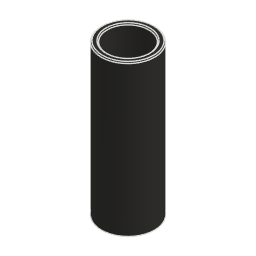
8mm_bearing_adapter_x2 (Autodesk Fusion 360 design; units mm, degrees)
Autodesk Fusion 360 part; units mm, degrees
sketch "Sketch1" plane through (0, 0, 0) normal (0, 1, 0) x (1, 0, 0)
  line L0 (0, 0) -> (0, -55)
  line L1 (0, -55) -> (-9.675, -55)
  line L2 (-9.675, -55) -> (-9.675, 0)
  line L3 (-9.675, 0) -> (0, 0)
  line L4 (-7.5, -55) -> (-7.5, -30.5)
  line L5 (-7.5, 0) -> (-7.5, -24.5)
  line L6 (-7.5, -24.5) -> (0, -24.5)
  line L7 (-7.5, -30.5) -> (0, -30.5)
  line L8 (-7.5, -24.5) -> (-7.5, -30.5)
  line L9 (-5.5, -24.5) -> (-5.5, -30.5)
  dimension "d1" = 19.35
  dimension "d2" = 55
  dimension "d5" = 24.5
  dimension "d6" = 24.5
  dimension "d7" = 15
  dimension "d27" = 2
  constraint coincident L0.start L3.end
  constraint vertical L0
  constraint vertical L2
  constraint horizontal L3
  constraint horizontal L1
  constraint coincident L1 L4.start
  constraint vertical L4
  constraint coincident L3 L5.start
  constraint vertical L5
  constraint coincident L0 L6.end
  constraint coincident L0 L7.end
  constraint horizontal L7
  constraint horizontal L6
  constraint coincident L7 L4.end
  constraint vertical L8
  constraint coincident L4.end L7.start
  constraint coincident L5.end L6.start
  constraint coincident L6 L9.start
  constraint coincident L7 L9.end
  constraint perpendicular L7 L9
  measures "d2" distance of L0.start L0.end
  measures "d5" distance of L5.start L5.end
  measures "d6" distance of L4.start L4.end
  measures "d27" distance of L4.end L9.end
revolve "Revolve1" add sketch "Sketch1" angle 360 about axis through (0, 0, 0) along (0, 0, 1) contours L1 L2 L3 L4 L5 L8 | L6 L7 L8 L9
move_face "OffsetFaces2" offset -0.075 3 faces at (-7.4627, 0.7468, 46.8333) (-7.4907, 0.3738, 16.3333) (-5.4932, 0.2742, 26.5)
chamfer "Chamfer5" distance 0.4 angle 45 2 edges at (7.0624, -2.7392, 55) (-9.0203, 3.4986, 55)
chamfer "Chamfer6" distance 0.2 angle 45 2 edges at (7.0624, -2.7392, 0) (-9.0203, 3.4986, 0)
chamfer "Chamfer7" distance 2 angle 45 2 edges at (5.1977, -2.016, 24.5) (5.1977, -2.016, 30.5)
equation "d6 = d5"
equation "tolerance = ( 0.15 / 2 ) * 1 mm"
equation "d28 = -tolerance"
